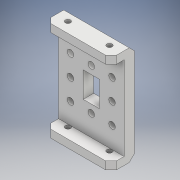
# Autodesk Inventor part: fixation_ax12
Saved by Autodesk Inventor 2017 (Build 210142000, 142)
## iProperties
Created: 2017-11-23
Part Number: fixation_ax12
Material: ABS Plastic
Document SubType Name: Modeling
Designer: Biscuit
Density: 1.06 g/cm^3
Appearance: Smooth - White
Author: Biscuit
Autodesk Inventor part; units mm, degrees
ref_plane "YZ Plane" through (0, 0, 0) normal (1, 0, 0) x (0, 1, 0)
ref_plane "XZ Plane" through (0, 0, 0) normal (0, 1, 0) x (-1, 0, 0)
ref_plane "XY Plane" through (0, 0, 0) normal (0, 0, 1) x (1, 0, 0)
sketch "Sketch1" plane through (0, 0, 0) normal (0, 1, 0) x (-1, 0, 0)
  line L0 (0, 0) -> (25.2, 0)
  line L1 (25.2, 0) -> (25.2, -32.2)
  line L2 (25.2, -32.2) -> (0, -32.2)
  line L3 (0, -32.2) -> (0, 0)
  line L4 (15.7, -11.2) -> (9.5, -11.2)
  line L5 (9.5, -11.2) -> (9.5, -21)
  line L6 (9.5, -21) -> (15.7, -21)
  line L7 (15.7, -21) -> (15.7, -11.2)
  circle A0 centre (20.6, -8.1) radius 1.25
  circle A1 centre (20.6, -16.1) radius 1.25
  circle A2 centre (20.6, -24.1) radius 1.25
  circle A3 centre (12.6, -8.1) radius 1.25
  circle A4 centre (12.6, -16.1) radius 1.25
  circle A5 centre (12.6, -24.1) radius 1.25
  circle A6 centre (4.6, -8.1) radius 1.25
  circle A7 centre (4.6, -16.1) radius 1.25
  circle A8 centre (4.6, -24.1) radius 1.25
  dimension "d0" = 25.2
  dimension "d1" = 32.2
  dimension "d2" = 9.5
  dimension "d3" = 9.5
  dimension "d4" = 11.2
  dimension "d5" = 11.2
  dimension "d6" = 2.5
  dimension "d9" = 8
  dimension "d12" = 8
  dimension "d15" = 4.6
  dimension "d16" = 4.6
  dimension "d17" = 16.1
  dimension "d18" = 16.1
  constraints: 16 end point, 9 centre point, 4 parallel, 3 horizontal, 2 perpendicular, 1 vertical, 16 other
  measures "d0" distance of L1.end L2.end
  measures "d1" distance of L0.end L1.end
  measures "d2" distance between parallel lines of L1 L7
  measures "d3" distance between parallel lines of L3 L5
  measures "d4" distance between parallel lines of L2 L6
  measures "d5" distance between parallel lines of L0 L4
  measures "d6" diameter of A0
  measures "d9" distance of A0.centre A1.centre
  measures "d12" distance of A0.centre A3.centre
  measures "d15" distance from line of L1 A0.centre
  measures "d16" distance from line of L3 A6.centre
  measures "d17" distance from line of L2 A1.centre
  measures "d18" distance from line of L0 A1.centre
extrude "Extrusion1" add sketch "Sketch1" along normal blind 4 contours L0 L1 L2 L3
sketch "Sketch2" plane through (-25.2, 0, 0) normal (0, 0, 1) x (1, 0, 0)
  line L0 (0, 0) -> (0, 4) projected
  line L1 (0, 4) -> (25.2, 4)
  line L2 (25.2, 4) -> (25.2, -5)
  line L3 (25.2, -5) -> (0, -5)
  line L4 (0, -5) -> (0, 4)
  circle A0 centre (4.6, -1) radius 1
  circle A1 centre (20.6, -1) radius 1
  point P0 (25.2, 0)
  dimension "d21" = 9
  dimension "d22" = 25.2
  dimension "d23" = 2
  dimension "d24" = 2
  dimension "d25" = 4.6
  dimension "d26" = 4.6
  dimension "d27" = 5
  dimension "d28" = 5
  constraints: 8 end point, 2 centre point, 2 parallel, 1 horizontal, 1 perpendicular
  measures "d21" distance of L3.end L0.end
  measures "d22" distance between parallel lines of L4 L2
  measures "d23" diameter of A0
  measures "d24" diameter of A1
  measures "d25" distance from line of L4 A0.centre
  measures "d26" distance from line of L2 A1.centre
  measures "d27" distance from line of L1 A0.centre
  measures "d28" distance from line of L1 A1.centre
extrude "Extrusion2" add sketch "Sketch2" along normal blind 3
sketch "Sketch3" plane through (0, 0, -32.2) normal (0, 0, -1) x (-1, 0, 0)
  line L0 (0, 0) -> (0, 4)
  line L1 (0, 4) -> (25.2, 4)
  line L2 (25.2, 4) -> (25.2, -5)
  line L3 (25.2, -5) -> (0, -5)
  line L4 (0, -5) -> (0, 4)
  circle A0 centre (4.6, -1) radius 1
  circle A1 centre (20.6, -1) radius 1
  point P0 (25.2, 0)
  dimension "d31" = 9
  dimension "d32" = 25.2
  dimension "d33" = 2
  dimension "d34" = 2
  dimension "d35" = 4.6
  dimension "d36" = 4.6
  dimension "d37" = 5
  dimension "d38" = 5
  constraints: 10 end point, 2 centre point, 2 parallel, 1 horizontal, 1 perpendicular
  measures "d31" distance of L3.end L0.end
  measures "d32" distance between parallel lines of L4 L2
  measures "d33" diameter of A0
  measures "d34" diameter of A1
  measures "d35" distance from line of L4 A0.centre
  measures "d36" distance from line of L2 A1.centre
  measures "d37" distance from line of L1 A0.centre
  measures "d38" distance from line of L1 A1.centre
extrude "Extrusion3" add sketch "Sketch3" along normal blind 3
chamfer "Chamfer1" distance 2 angle 45 6 edges at (-12.6, 4, -35.2) (-12.6, 4, 3) (0, -5, 1.5) (-25.2, -5, 1.5) (-25.2, -5, -33.7) (0, -5, -33.7)
equation "\"d3\" = d2"
equation "\"d5\" = d4"
equation "\"d15\" = d16"
equation "\"d17\" = d18"
equation "\"d24\" = d23"
equation "\"d26\" = d25"
equation "\"d28\" = d27"
equation "\"d34\" = d33"
equation "\"d36\" = d35"
equation "\"d38\" = d37"
body "Solid1"
